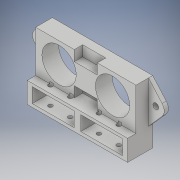
# Autodesk Inventor part: FrontSensor
Saved by Autodesk Inventor 2019 (Build 230136000, 136)
## iProperties
Created: 2021-01-02
Part Number: FrontSensor
Material: Типовые
Document SubType Name: Modeling
Designer: Professional
Density: 1 g/cm^3
Appearance: По умолчанию
Author: Professional
Autodesk Inventor part; units mm, degrees
ref_plane "YZ Plane" through (0, 0, 0) normal (1, 0, 0) x (0, 1, 0)
ref_plane "XZ Plane" through (0, 0, 0) normal (0, 1, 0) x (-1, 0, 0)
ref_plane "XY Plane" through (0, 0, 0) normal (0, 0, 1) x (1, 0, 0)
sketch "Эскиз1" plane through (0, 0, 0) normal (0, 0, 1) x (1, 0, 0)
  line L0 (-24, 10) -> (24, 10)
  line L1 (24, 10) -> (24, -10) construction
  line L2 (24, -10) -> (-24, -10)
  line L3 (-24, -10) -> (-24, 10) construction
  line L4 (0, 10) -> (0, -10)
  arc A0 (-30.4971, 2.649) -> (-30.4971, -2.649) centre (-27.5, 0) ccw
  line L5 (-30.4971, 2.649) -> (-24, 10)
  line L6 (-30.4971, -2.649) -> (-24, -10)
  arc A1 (30.4971, -2.649) -> (30.4971, 2.649) centre (27.5, 0) ccw
  line L7 (30.4971, 2.649) -> (24, 10)
  line L8 (30.4971, -2.649) -> (24, -10)
  point P0 (0, 0)
  point P1 (0, 0)
  dimension "d0" = 20
  dimension "d1" = 48
  dimension "d2" = 4
  dimension "d3" = 55
  constraints: 18 end point, 4 point on circle, 3 midpoint, 3 symmetric about line, 2 centre point, 2 parallel, 2 tangent, 1 coincident, 1 equal length, 1 horizontal, 1 perpendicular, 1 other
  measures "d0" distance between parallel lines of L0 L2
  measures "d1" distance between parallel lines of L1 L3
  measures "d2" radius of A0
  measures "d3" diameter of A0.centre L4
extrude "Выдавливание1" add sketch "Эскиз1" along normal blind 2
sketch "Эскиз2" plane through (0, 0, 2) normal (0, 0, 1) x (1, 0, 0)
  line L0 (24, 10) -> (-24, 10) projected
  line L1 (24, -10) -> (30.4971, -2.649) projected
  line L2 (-24, 10) -> (24, 10)
  line L3 (24, 10) -> (24, -10)
  line L4 (24, -10) -> (-24, -10)
  line L5 (-24, -10) -> (-24, 10)
  point P0 (0, 0)
  constraints: 8 end point, 2 parallel, 1 horizontal, 1 perpendicular
extrude "Выдавливание2" add sketch "Эскиз2" along normal blind 6
sketch "Эскиз3" plane through (0, 0, 8) normal (0, 0, 1) x (1, 0, 0)
  circle A0 centre (-12.8, 0) radius 8.2
  circle A1 centre (12.8, 0) radius 8.2
  line L0 (-24, -10) -> (24, -10) projected
  line L1 (0, -10) -> (0, 10)
  line L2 (24, 10) -> (-24, 10) projected
  point P0 (0, 0)
  dimension "d8" = 25.6
  dimension "d9" = 16.4
  constraints: 2 centre point, 2 end point, 2 midpoint, 1 horizontal alignment, 1 other
  measures "d8" distance of A1.centre A0.centre
  measures "d9" diameter of A1
extrude "Выдавливание3" cut sketch "Эскиз3" against normal through all
sketch "Эскиз4" plane through (0, 0, 8) normal (0, 0, 1) x (1, 0, 0)
  line L0 (24, 10) -> (-24, 10) projected
  line L1 (-5.5, 10) -> (5.5, 10)
  line L2 (5.5, 10) -> (5.5, 5)
  line L3 (5.5, 5) -> (-5.5, 5)
  line L4 (-5.5, 5) -> (-5.5, 10)
  line L5 (-24, 10) -> (-24, -10) construction
  line L6 (-24, 0) -> (24, 0)
  line L7 (24, -10) -> (24, 10) construction
  line L8 (-5.5, -10) -> (5.5, -10)
  line L9 (5.5, -10) -> (5.5, -5)
  line L10 (5.5, -5) -> (-5.5, -5)
  line L11 (-5.5, -5) -> (-5.5, -10)
  point P0 (0, 0)
  point P1 (0, 0)
  point P2 (0, 5)
  point P3 (0, -5)
  dimension "d12" = 5
  dimension "d13" = 11
  constraints: 18 end point, 5 symmetric about line, 4 midpoint, 2 parallel, 1 horizontal, 1 perpendicular, 1 point on line, 1 vertical alignment
  measures "d12" distance between parallel lines of L0 L3
  measures "d13" distance between parallel lines of L2 L4
extrude "Выдавливание4" cut sketch "Эскиз4" against normal blind 4
sketch "Эскиз5" plane through (0, 0, 2) normal (0, 0, 1) x (1, 0, 0)
  arc A0 (-30.4971, 2.649) -> (-30.4971, -2.649) centre (-27.5, 0) ccw projected
  arc A1 (30.4971, -2.649) -> (30.4971, 2.649) centre (27.5, 0) ccw projected
  point P0 (0, 0)
  point P1 (27.5, 0)
  constraints: 2 coincident
hole "Отверстие1" at (-27.5, 0, 2) at (27.5, 0, 2) direction (0, 0, -1) diameter 2.8 end through all
sketch "Эскиз6" plane through (0, 0, 0) normal (0, 0, -1) x (-1, 0, 0)
  line L0 (24, -10) -> (-24, -10) projected
  line L1 (24, -10) -> (-24, -10)
  line L2 (-24, -10) -> (-24, -20)
  line L3 (-24, -20) -> (24, -20)
  line L4 (24, -20) -> (24, -10)
  line L5 (-5.5, -10) -> (5.5, -10) projected
  line L6 (0, -20) -> (0, -10)
  line L7 (21.6, -18.4) -> (1.6, -18.4)
  line L8 (1.6, -18.4) -> (1.6, -11.4)
  line L9 (1.6, -11.4) -> (21.6, -11.4)
  line L10 (21.6, -11.4) -> (21.6, -18.4)
  line L11 (-1.6, -11.4) -> (-21.6, -11.4)
  line L12 (-21.6, -11.4) -> (-21.6, -18.4)
  line L13 (-21.6, -18.4) -> (-1.6, -18.4)
  line L14 (-1.6, -18.4) -> (-1.6, -11.4)
  point P0 (0, 0)
  point P1 (0, -10)
  dimension "d25" = 10
  dimension "d26" = 48
  dimension "d41" = 20
  dimension "d42" = 7
  dimension "d43" = 1.6
  dimension "d44" = 3.2
  constraints: 26 end point, 6 parallel, 4 perpendicular, 3 horizontal, 3 midpoint, 3 point on line, 1 vertical alignment, 2 other
  measures "d25" distance between parallel lines of L0 L3
  measures "d26" distance between parallel lines of L4 L2
  measures "d41" distance between parallel lines of L8 L10
  measures "d42" distance between parallel lines of L7 L9
  measures "d43" distance between parallel lines of L3 L7
  measures "d44" distance between parallel lines of L14 L8
extrude "Выдавливание5" add sketch "Эскиз6" against normal blind 12
sketch "Эскиз7" plane through (-24, -20, 0) normal (0, -1, 0) x (1, 0, 0)
  line L0 (24, 0) -> (24, 12)
  line L1 (48, 0) -> (0, 0) projected
  line L2 (48, 0) -> (0, 0) projected
  line L3 (48, 0) -> (48, 12) projected
  line L4 (0, 12) -> (48, 12) projected
  line L5 (0, 0) -> (0, 12) projected
  line L6 (45.6, 0) -> (25.6, 0) projected
  line L7 (45.6, 0) -> (45.6, 12) projected
  line L8 (25.6, 12) -> (45.6, 12) projected
  line L9 (25.6, 0) -> (25.6, 12) projected
  line L10 (22.4, 0) -> (2.4, 0) projected
  line L11 (22.4, 0) -> (22.4, 12) projected
  line L12 (2.4, 12) -> (22.4, 12) projected
  line L13 (2.4, 0) -> (2.4, 12) projected
  line L14 (0, 12) -> (48, 12) projected
  line L15 (12.4, 12) -> (12.4, 0)
  line L16 (45, 0) -> (28.6, 0) projected
  line L17 (35.6, 0) -> (35.6, 12)
  point P0 (7.65, 8.6)
  point P1 (17.15, 8.6)
  point P2 (30.85, 8.6)
  point P3 (40.35, 8.6)
  dimension "d46" = 9.5
  dimension "d47" = 8.6
  constraints: 6 end point, 3 midpoint, 3 symmetric about line, 2 horizontal alignment, 2 point on line, 2 vertical
  measures "d46" distance of point (7.65, 8.6) point (17.15, 8.6)
  measures "d47" distance from line of L1 point (17.15, 8.6)
hole "Отверстие2" at (-16.35, -20, 8.6) at (-6.85, -20, 8.6) at (6.85, -20, 8.6) at (16.35, -20, 8.6) direction (0, 1, 0) diameter 2 depth 11
